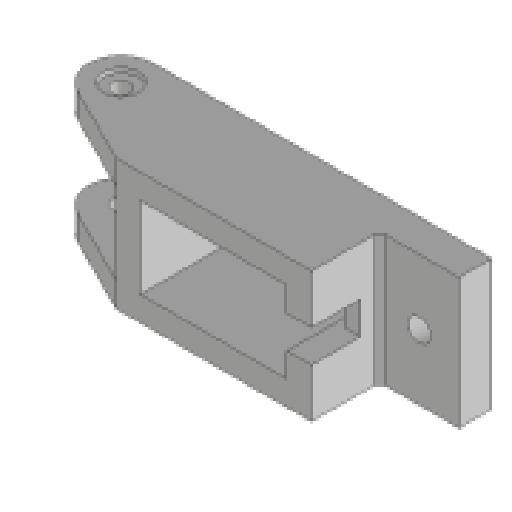
# Autodesk Inventor part: Servo Base
Saved by Autodesk Inventor 2025 (Build 290162010, 162A)
## iProperties
Created: 2024-11-29
Part Number: Servo Base
Material: Generic
Document SubType Name: Modeling
Designer: alexa
Density: 1 g/cm^3
Appearance: Default
Author: alexa
Autodesk Inventor part; units mm, degrees
ref_plane "YZ Plane" through (0, 0, 0) normal (1, 0, 0) x (0, 1, 0)
sketch "Sketch1" plane through (0, 0, 0) normal (0, 0, 1) x (1, 0, 0)
  line L0 (0, 0) -> (22.86, 0)
  line L1 (22.86, 0) -> (22.86, 12.7)
  line L2 (22.86, 12.7) -> (0, 12.7)
  line L3 (0, 12.7) -> (0, 0)
  line L4 (-3.81, 16.51) -> (26.67, 16.51)
  line L5 (26.67, 16.51) -> (26.67, -3.81)
  line L6 (26.67, -3.81) -> (-3.81, -3.81)
  line L7 (-3.81, -3.81) -> (-3.81, 16.51)
  dimension "d0" = 22.86
  dimension "d1" = 12.7
  dimension "d2" = 20.32
  constraints: 16 end point, 4 parallel, 2 perpendicular, 1 horizontal, 3 other
  measures "d0" distance of L0.start L0.end
  measures "d1" distance of L2.end L0.start
  measures "d2" distance between parallel lines of L4 L6
extrude "Extrusion1" add sketch "Sketch1" along normal blind 15.6972
sketch "Sketch2" plane through (26.67, -3.81, 0) normal (1, 0, 0) x (0, 0, -1)
  line L0 (-15.6972, 16.51) -> (-15.6972, 3.81) projected
  line L1 (-15.6972, 12.7) -> (-8.0772, 12.7)
  line L2 (-8.0772, 12.7) -> (-8.0772, 7.62)
  line L3 (-8.0772, 7.62) -> (-15.6972, 7.62)
  line L4 (-15.6972, 7.62) -> (-15.6972, 12.7)
  line L5 (0, 0) -> (0, 20.32) projected
  point P0 (0, 3.81)
  point P1 (-8.0772, 10.16)
  point P2 (0, 10.16)
  dimension "d5" = 5.08
  dimension "d6" = 7.62
  constraints: 8 end point, 2 midpoint, 2 parallel, 1 horizontal, 1 horizontal alignment, 1 perpendicular, 1 point on line
  measures "d5" distance of L1.end L2.end
  measures "d6" distance of L2.end L3.end
extrude "Extrusion2" cut sketch "Sketch2" against normal up to surface (3.81 mm away)
sketch "Sketch3" plane through (0, 0, 0) normal (0, 0, -1) x (-1, 0, 0)
  line L0 (3.81, -3.81) -> (-26.67, -3.81) projected
  line L1 (3.81, -3.81) -> (4.7498, -3.81)
  line L2 (4.7498, -3.81) -> (4.7498, 16.51)
  line L3 (4.7498, 16.51) -> (3.81, 16.51)
  line L4 (3.81, 16.51) -> (3.81, -3.81)
  line L5 (0, 0) -> (0, 12.7) projected
  line L6 (-26.67, -3.81) -> (-27.6098, -3.81)
  line L7 (-27.6098, -3.81) -> (-27.6098, 16.51)
  line L8 (-27.6098, 16.51) -> (-26.67, 16.51)
  line L9 (-26.67, 16.51) -> (-26.67, -3.81)
  line L10 (-22.86, 12.7) -> (-22.86, 0) projected
  dimension "d9" = 4.7498
  dimension "d18" = 4.7498
  constraints: 16 end point, 4 parallel, 2 coincident, 2 horizontal, 2 perpendicular
  measures "d9" distance between parallel lines of L2 L5
  measures "d18" distance between parallel lines of L10 L7
extrude "Extrusion3" add sketch "Sketch3" against normal blind 5.08
chamfer "Chamfer1" distance 0.9398 angle 45 2 edges at (-3.81, 6.35, 5.08) (26.67, 6.35, 5.08)
sketch "Sketch4" plane through (0, 0, 0) normal (0, 0, -1) x (-1, 0, 0)
  circle A0 centre (2.54, 6.35) radius 0.889
  line L0 (4.7498, -3.81) -> (3.81, -3.81) construction
  line L1 (0, 0) -> (4.7498, 0) construction
  line L2 (4.7498, 0) -> (4.7498, -3.81) construction
  line L3 (4.7498, -3.81) -> (0, -3.81) construction
  line L4 (0, -3.81) -> (0, 0) construction
  line L5 (4.7498, -3.81) -> (4.7498, 16.51) projected
  line L6 (-22.86, 0) -> (0, 0) projected
  line L7 (-11.43, 0) -> (-11.43, 12.7) construction
  line L8 (0, 12.7) -> (-22.86, 12.7) projected
  circle A1 centre (-25.4, 6.35) radius 0.889
  point P0 (2.3749, -3.81)
  point P1 (4.7498, 6.35)
  dimension "d15" = 1.778
  dimension "d27" = 13.97
  constraints: 10 end point, 4 midpoint, 2 centre point, 2 parallel, 1 horizontal, 1 horizontal alignment, 1 perpendicular, 1 symmetric about line, 1 other
  measures "d15" diameter of A0
  measures "d27" distance from line of L7 A0.centre
extrude "Extrusion4" cut sketch "Sketch4" against normal blind 7.62
ref_plane "Work Plane1" through (11.43, -3.81, 15.6972) normal (-1, 0, 0) x (0, 0, 1)
sketch "Sketch5" plane through (-3.81, 16.51, 15.6972) normal (0, 1, 0) x (1, 0, 0)
  line L0 (0, 0) -> (30.48, 0) projected
  line L1 (-0.9398, 15.6972) -> (-0.9398, 10.6172) projected
  line L2 (0, 9.6774) -> (-0.9398, 10.6172) projected
  line L3 (0, 9.6774) -> (0, 0) projected
  line L4 (-0.9398, 15.6972) -> (31.4198, 15.6972) projected
  line L5 (-0.9398, 15.6972) -> (-7.1489, 19.555)
  line L6 (-13.1566, 11.4009) -> (0, 0)
  arc A0 (-7.1489, 19.555) -> (-13.1566, 11.4009) centre (-9.8298, 15.24) ccw
  circle A1 centre (-9.8298, 15.24) radius 1.397
  line L7 (-0.9398, 10.6172) -> (0, 9.6774) projected
  point P0 (3.81, 15.6972)
  dimension "d24" = 5.08
  dimension "d25" = 8.89
  dimension "d26" = 2.794
  dimension "d42" = 15.24
  constraints: 4 end point, 2 centre point, 2 point on circle, 2 tangent, 1 coincident
  measures "d24" radius of A0
  measures "d25" distance from line of L1 A0.centre
  measures "d26" diameter of A1
  measures "d42" distance from line of A0.centre L0
extrude "Extrusion5" add sketch "Sketch5" against normal blind 3.81
ref_plane "Work Plane2" through (26.67, 6.35, 15.6972) normal (0, 1, 0) x (1, 0, 0)
mirror "Mirror1" about plane through (26.67, 6.35, 15.6972) normal (0, 1, 0) of "Extrusion5"
sketch "Sketch6" plane through (27.6098, 16.51, 5.08) normal (0, 1, 0) x (1, 0, 0)
  circle A0 centre (-41.2496, 4.6228) radius 1.397 projected
  circle A1 centre (-41.2496, 4.6228) radius 2.794
  point P0 (-27.6098, 5.08)
  dimension "d29" = 5.588
  constraints: 1 centre point, 1 coincident
  measures "d29" diameter of A1
extrude "Extrusion6" cut sketch "Sketch6" against normal blind 0.762
mirror "Mirror2" about plane through (26.67, 6.35, 15.6972) normal (0, 1, 0) of "Extrusion6"
sketch "Sketch7" plane through (27.6098, -3.81, 0) normal (1, 0, 0) x (0, 0, -1)
  line L0 (0, 20.32) -> (0, 0) projected
  line L1 (0, 20.32) -> (-5.08, 20.32) projected
  line L2 (-5.08, 0) -> (-5.08, 20.32) projected
  line L3 (0, 0) -> (-5.08, 0) projected
  point P0 (0, 3.81)
extrude "Extrusion7" add sketch "Sketch7" along normal blind 11.43
sketch "Sketch8" plane through (0, 0, 0) normal (0, 0, -1) x (-1, 0, 0)
  circle A0 centre (-32.8549, 6.35) radius 1.778
  line L0 (-39.0398, -3.81) -> (-39.0398, 16.51) projected
  line L1 (-26.67, 16.51) -> (-26.67, -3.81) projected
  line L2 (10.9589, 16.51) -> (-39.0398, 16.51) projected
  line L3 (-26.67, 16.51) -> (-39.0398, 16.51)
  point P0 (0, 0)
  point P1 (-39.0398, 6.35)
  point P2 (-32.8549, 16.51)
  dimension "d34" = 3.556
  constraints: 2 end point, 2 midpoint, 1 centre point, 1 collinear, 1 horizontal alignment, 1 vertical alignment
  measures "d34" diameter of A0
extrude "Extrusion8" cut sketch "Sketch8" against normal blind 18.7325
sketch "Sketch9" plane through (0, 0, 0) normal (0, 0, -1) x (-1, 0, 0)
  line L0 (-22.86, 12.7) -> (-22.86, 0) projected
  line L1 (-22.86, 3.81) -> (-24.257, 3.81)
  line L2 (-24.257, 3.81) -> (-24.257, 8.89)
  line L3 (-24.257, 8.89) -> (-22.86, 8.89)
  line L4 (-22.86, 8.89) -> (-22.86, 3.81)
  point P0 (0, 0)
  point P1 (-22.86, 6.35)
  dimension "d37" = 5.08
  dimension "d38" = 1.397
  dimension "d39" = 2.54
  constraints: 8 end point, 2 parallel, 1 horizontal, 1 midpoint, 1 perpendicular, 1 point on line
  measures "d37" distance of L1.end L2.end
  measures "d38" distance between parallel lines of L0 L2
  measures "d39" distance from line of point (-22.86, 6.35) L1
extrude "Extrusion9" cut sketch "Sketch9" against normal blind 22.225
equation "\"d18\" = d9"
equation "\"d39\" = 0.5 * d37"
body "Solid1"
